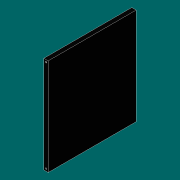
# Autodesk Inventor part: sides
Saved by Autodesk Inventor 2016 (Build 200138000, 138)
## iProperties
Created: 2015-10-13
Part Number: sides
Material: PC/ABS Plastic
Document SubType Name: Modeling
Designer: Sawaiz
Density: 0.357273 g/cm^3
Appearance: Smooth - Black
Author: Sawaiz
Autodesk Inventor part; units mm, degrees
ref_plane "YZ Plane" through (0, 0, 0) normal (1, 0, 0) x (0, 1, 0)
ref_plane "XZ Plane" through (0, 0, 0) normal (0, 1, 0) x (-1, 0, 0)
ref_plane "XY Plane" through (0, 0, 0) normal (0, 0, 1) x (1, 0, 0)
sketch "Sketch1" plane through (0, 0, 0) normal (0, 1, 0) x (-1, 0, 0)
  line L0 (-73.025, 69.85) -> (73.025, 69.85)
  line L1 (73.025, 69.85) -> (73.025, -69.85)
  line L2 (73.025, -69.85) -> (-73.025, -69.85)
  line L3 (-73.025, -69.85) -> (-73.025, 69.85)
  line L4 (-73.025, 69.85) -> (73.025, -69.85) construction
  line L5 (73.025, 69.85) -> (-73.025, -69.85) construction
  point P0 (0, 0)
  dimension "d0" = 146.05
  dimension "d1" = 139.7
  constraints: 12 end point, 2 midpoint, 2 parallel, 1 horizontal, 1 perpendicular
  measures "d0" distance of L1.end L2.end
  measures "d1" distance of L0.end L1.end
extrude "Extrusion1" add sketch "Sketch1" along normal blind 6.35
sketch "Sketch9" plane through (73.025, 0, 69.85) normal (1, 0, 0) x (0, 0, -1)
  line L0 (139.7, 0) -> (0, 0) projected
  line L1 (139.7, 0) -> (139.7, 6.35) projected
  line L2 (0, 6.35) -> (139.7, 6.35) projected
  line L3 (0, 0) -> (0, 6.35) projected
  point P0 (69.85, 0)
  point P1 (3.175, 3.175)
  dimension "d45" = 3.175
  dimension "d46" = 3.175
  measures "d45" distance from line of L0 point (3.175, 3.175)
  measures "d46" distance from line of L3 point (3.175, 3.175)
hole "Hole3" at (73.025, 3.175, 66.675) direction (-1, 0, 0) diameter 2.156 depth 8.865 tip angle 118 thread size "4-40 UNC" class "2B" standard "ANSI Unified Screw Threads"
mirror "Mirror5" about plane through (0, 0, 0) normal (0, 0, 1) of "Hole3"
mirror "Mirror6" about plane through (0, 0, 0) normal (1, 0, 0) of "Hole3", "Mirror5"
sketch "Sketch10" plane through (0, 0, 0) normal (0, -1, 0) x (1, 0, 0)
  line L0 (73.025, 69.85) -> (-73.025, 69.85) projected
  line L1 (-73.025, 69.85) -> (-73.025, -69.85) projected
  line L2 (-73.025, -69.85) -> (73.025, -69.85) projected
  line L3 (73.025, -69.85) -> (73.025, 69.85) projected
  line L4 (34.1313, -65.0875) -> (35.7188, -65.0875)
  line L5 (35.7188, -65.0875) -> (35.7187, 65.0875)
  line L6 (35.7187, 65.0875) -> (34.1312, 65.0875)
  line L7 (34.1312, 65.0875) -> (34.1313, -65.0875)
  point P0 (0, 0)
  dimension "d54" = 1.5875
  dimension "d55" = 37.3062
  dimension "d56" = 4.7625
  dimension "d57" = 4.7625
  constraints: 8 end point, 2 parallel, 1 horizontal, 1 perpendicular
  measures "d54" distance between parallel lines of L5 L7
  measures "d55" distance between parallel lines of L3 L5
  measures "d56" distance between parallel lines of L0 L6
  measures "d57" distance between parallel lines of L2 L4
extrude "Extrusion6" cut sketch "Sketch10" against normal blind 1.5875 contours L7 L6 L5 L4
fillet "Fillet2" radius 0.7937 4 edges at (35.7187, 0.7937, 65.0875) (34.1312, 0.7937, 65.0875) (35.7188, 0.7937, -65.0875) (34.1313, 0.7937, -65.0875)
equation "\"d0\" = depth"
equation "\"d1\" = height + 2 * plasticThickness"
equation "\"d2\" = plasticThickness"
equation "\"d45\" = 0.5 * plasticThickness"
equation "\"d46\" = 0.5 * plasticThickness"
equation "\"d55\" = aerogelHolderDepth"
equation "\"d58\" = 0.25 * plasticThickness"
equation "\"acrylicThickness\" = 9.525"
equation "\"depth\" = 146.05"
equation "\"height\" = 127"
equation "\"fresnelThickness\" = 0.1"
equation "\"focalLength\" = 76.2"
equation "\"centerThickness\" = 1.524"
equation "\"sensorHolderDepth\" = 19.05"
equation "\"internalAcrylicThickness\" = 6.35"
equation "\"frameAcrylicThickness\" = 9.525"
equation "\"width\" = 127"
equation "\"mirrorAngle\" = 5deg"
equation "\"detectorWidth\" = 52"
equation "\"detectorHeight\" = 52"
equation "\"mirrorThickness\" = 3.175"
equation "\"ior\" = 1.49"
equation "\"fresnelAngle\" = 90deg"
equation "\"fresnelEffectiveDiameter\" = 152.4"
equation "\"oRingWidth\" = 1.5875"
equation "\"aerogelClearence\" = 3.175"
equation "\"backplanePCBHeight\" = 76.2"
equation "\"backplaneHoleOffsett\" = 6.35"
equation "\"backplanePCBWidth\" = 76.2"
equation "\"backplanePostionOffsett\" = 12.7"
equation "\"moduleSlotClearence\" = 0.79375"
equation "\"plasticThickness\" = 6.35"
equation "\"aerogelHolderDepth\" = 37.30625"
body "Solid1"
